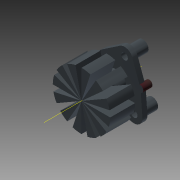
# Autodesk Inventor part: motor_GM1806-80T_SkyproRO
Saved by Autodesk Inventor 2015 SP1 (Build 190203100, 203)
## iProperties
Created: 2015-08-06
Part Number: motor_GM1806-80T_SkyproRO
Material: Iron, Cast
Document SubType Name: Modeling
Designer: Alexandre Cherpillod
Density: 7.15 g/cm^3
Appearance: Iron Gray
Mass: 11.1743 g
Surface Area: 29.2537 cm^2
Volume: 1.56283 cm^3
Author: Alexandre Cherpillod
Autodesk Inventor part; units mm, degrees
ref_plane "YZ Plane" through (0, 0, 0) normal (1, 0, 0) x (0, 1, 0)
ref_plane "XZ Plane" through (0, 0, 0) normal (0, 1, 0) x (-1, 0, 0)
sketch "Sketch1" plane through (0, 0, 0) normal (0, 1, 0) x (-1, 0, 0)
  arc A0 (0, -8.65) -> (2.673, -8.2266) centre (0, 0) ccw
  line L0 (0, 0) -> (2.673, -8.2266) construction
  line L1 (0, 0) -> (0, -8.65) construction
  line L2 (0, 0) -> (2.673, -8.2266)
  line L3 (0, -8.65) -> (0, 0)
  dimension "d0" = 8.65
  dimension "d1" = 18
  constraints: 8 end point, 2 collinear, 2 point on circle, 1 centre point, 1 coincident
  measures "d0" radius of A0
  measures "d1" angle of L1 L0
extrude "Extrusion1" add sketch "Sketch1" along normal blind 7.5
pattern_circular "Circular Pattern1" count 12 over 360 about axis through (0, -10, 0) along (0, 1, 0) of "Extrusion1"
ref_plane "Work Plane1" through (-8.461, 12, -1.7984) normal (0, 1, 0) x (0.9781, 0, 0.2079)
sketch "Sketch2" plane through (-8.461, 12, -1.7984) normal (0, 1, 0) x (0.9781, 0, 0.2079)
  line L0 (8.65, 0) -> (0, 0) projected
  circle A0 centre (0.65, 0) radius 2.5
  circle A1 centre (12.65, -6.9282) radius 2.5
  circle A2 centre (12.65, 6.9282) radius 2.5
  line L1 (5.859, 6.8666) -> (11.7086, 9.2442)
  line L2 (15.1264, 7.271) -> (15.9921, 1.0162)
  line L3 (15.9921, -1.0162) -> (15.1264, -7.271)
  line L4 (11.7086, -9.2442) -> (5.859, -6.8666)
  line L5 (4.325, -7.4911) -> (8.65, 0) projected
  line L6 (4.0989, -5.8503) -> (-0.885, -1.9732)
  line L7 (-0.885, 1.9732) -> (4.0989, 5.8503)
  arc A3 (15.9921, -1.0162) -> (15.9921, 1.0162) centre (8.65, 0) ccw
  arc A4 (5.859, 6.8666) -> (4.0989, 5.8503) centre (8.65, 0) ccw
  arc A5 (4.0989, -5.8503) -> (5.859, -6.8666) centre (8.65, 0) ccw
  point P0 (15.1264, 7.271)
  point P1 (-0.885, 1.9732)
  dimension "d9" = 5
  dimension "d12" = 360
  dimension "d23" = 8
  constraints: 14 point on circle, 12 end point, 12 tangent, 10 coincident, 6 centre point, 1 point on line, 7 other
  measures "d9" diameter of A0
  measures "d23" distance of A3.centre A0.centre
extrude "Extrusion2" add sketch "Sketch2" against normal blind 1.5
sketch "Sketch3" plane through (-8.461, 12, -1.7984) normal (0, 1, 0) x (0.9781, 0, 0.2079)
  circle A0 centre (8.65, 0) radius 3
  dimension "d16" = 6
  constraints: 1 centre point, 1 coincident
  measures "d16" diameter of A0
extrude "Extrusion3" add sketch "Sketch3" against normal up to surface (4.5 mm away)
sketch "Sketch4" plane through (-8.461, 12, -1.7984) normal (0, 1, 0) x (0.9781, 0, 0.2079)
  line L0 (8.65, 0) -> (0, 0) projected
  circle A0 centre (0.65, 0) radius 1.725
  dimension "d19" = 3.45
  dimension "d20" = 8
  constraints: 1 centre point, 1 point on line
  measures "d19" diameter of A0
  measures "d20" distance of L0.start A0.centre
extrude "Extrusion4" add sketch "Sketch4" along normal blind 4
hole "Hole1" at (-7.8252, 16, -1.6633) direction (0, -1, 0) diameter 2 depth 8 tip angle 118
pattern_circular "Circular Pattern2" count 3 over 360 about axis through (0, -10, 0) along (0, 1, 0) of "Extrusion4", "Hole1"
sketch "Sketch5" plane through (-8.461, 12, -1.7984) normal (0, 1, 0) x (0.9781, 0, 0.2079)
  line L0 (8.65, 0) -> (17.3, 0) projected
  circle A0 centre (15.95, 0) radius 1
  dimension "d36" = 2
  dimension "d37" = 7.3
  constraints: 1 centre point, 1 point on line
  measures "d36" diameter of A0
  measures "d37" distance of L0.start A0.centre
extrude "Extrusion5" add sketch "Sketch5" along normal blind 1.25 and the other way blind 1.5
sketch "Sketch6" plane through (-8.461, 12, -1.7984) normal (0, 1, 0) x (0.9781, 0, 0.2079)
  circle A0 centre (8.65, 0) radius 2
  circle A1 centre (8.65, 0) radius 1.5
  dimension "d42" = 4
  dimension "d43" = 3
  constraints: 2 centre point, 2 coincident
  measures "d42" diameter of A0
  measures "d43" diameter of A1
extrude "Extrusion6" add sketch "Sketch6" along normal blind 2.3
body "Solid1"
